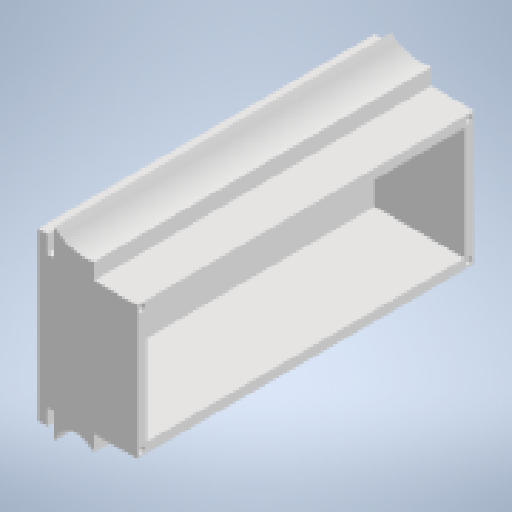
# Autodesk Inventor part: Casing
Saved by Autodesk Inventor 2025.2 (Build 292293000, 293)
## iProperties
Created: 2025-01-21
Part Number: Casing
Material: Generic
Document SubType Name: Modeling
Designer: armenanzasn25
Density: 1 g/cm^3
Appearance: Default
TUBE_OUTER: 0.545 in
Author: armenanzasn25
Autodesk Inventor part; units mm, degrees
ref_plane "YZ Plane" through (0, 0, 0) normal (1, 0, 0) x (0, 1, 0)
ref_plane "XZ Plane" through (0, 0, 0) normal (0, 1, 0) x (-1, 0, 0)
ref_plane "XY Plane" through (0, 0, 0) normal (0, 0, 1) x (1, 0, 0)
sketch "Sketch2" plane through (0, 0, 0) normal (0, 0, 1) x (1, 0, 0)
  line L0 (-3, 8) -> (-3, -48)
  line L1 (-3, 8) -> (3, 8)
  line L2 (3, 8) -> (3, 3)
  line L3 (3, 3) -> (5, 3)
  line L4 (5, 3) -> (5, 10.4583)
  arc A0 (5, 10.4583) -> (17, 10.4583) centre (11, 13.909) ccw
  line L5 (17, 10.4583) -> (17, 3)
  line L6 (17, 3) -> (27, 3)
  line L7 (-3, -48) -> (3, -48)
  line L8 (3, -43) -> (3, -48)
  line L9 (27, -43) -> (17, -43)
  arc A1 (17, -50.4583) -> (5, -50.4583) centre (11, -53.909) ccw
  line L10 (3, -43) -> (5, -43)
  line L11 (5, -43) -> (5, -50.4583)
  line L12 (17, -43) -> (17, -50.4583)
  line L13 (27, 3) -> (27, 0)
  line L14 (27, 0) -> (0, 0)
  line L15 (0, 0) -> (0, -40)
  line L16 (0, -40) -> (27, -40)
  line L17 (27, -40) -> (27, -43)
  dimension "d13" = 12
  dimension "d14" = 2
  dimension "d20" = 5
  dimension "d22" = 13.843
  dimension "d29" = 3
  dimension "d30" = 3
  dimension "d31" = 3
  dimension "d33" = 40
  dimension "d34" = 27
  dimension "d36" = 16
  dimension "d38" = 67.818
  dimension "d53" = 6.9215
  dimension "d54" = 10
  constraints: 36 end point, 8 perpendicular, 5 equal length, 4 point on circle, 4 vertical, 3 horizontal, 2 centre point, 2 collinear, 2 point on line, 1 coincident, 1 vertical alignment
  measures "d13" distance between parallel lines of L5 L4
  measures "d14" distance of L2.end L3.end
  measures "d20" distance between parallel lines of L1 L3
  measures "d22" diameter of A1
  measures "d29" distance between parallel lines of L6 L14
  measures "d30" distance between parallel lines of L0 L15
  measures "d31" distance between parallel lines of L9 L16
  measures "d33" distance between parallel lines of L16 L14
  measures "d34" distance of L13.end L14.end
  measures "d36" distance from line of L13 A0.centre
  measures "d38" distance of A1.centre A0.centre
  measures "d53" radius of A0
  measures "d54" distance between parallel lines of L13 L5
extrude "Extrusion1" add sketch "Sketch2" along normal blind 101.6
sketch "Sketch3" plane through (0, -40, 0) normal (1, 0, 0) x (0, 0, -1)
  line L0 (0, 0) -> (0, 40) projected
  line L1 (0, 40) -> (-101.6, 40) projected
  line L2 (-101.6, 0) -> (-101.6, 40) projected
  line L3 (0, 0) -> (-101.6, 0) projected
  line L4 (-101.6, 40) -> (-98.6, 40)
  line L5 (-98.6, 40) -> (-98.6, 0)
  line L6 (-98.6, 0) -> (-101.6, 0)
  line L7 (-101.6, 0) -> (-101.6, 40)
  line L8 (0, 40) -> (-3, 40)
  line L9 (-3, 40) -> (-3, 0)
  line L10 (-3, 0) -> (0, 0)
  line L11 (0, 0) -> (0, 40)
  dimension "d39" = 3
  dimension "d40" = 3
  constraints: 16 end point, 4 parallel, 2 horizontal, 2 perpendicular, 2 point on line
  measures "d39" distance between parallel lines of L5 L2
  measures "d40" distance between parallel lines of L0 L9
extrude "Extrusion2" add sketch "Sketch3" along normal blind 27 contours L3 L9 L1 L0 | L3 L2 L1 L5
sketch "Sketch4" plane through (27, -43, 0) normal (1, 0, 0) x (0, 0, -1)
  circle A0 centre (-100.1, 44.5) radius 1
  line L0 (-3, 3) -> (-98.6, 3) projected
  line L1 (-98.6, 3) -> (-98.6, 43) projected
  line L2 (-3, 43) -> (-98.6, 43) projected
  line L3 (-3, 43) -> (-3, 3) projected
  line L4 (0, 0) -> (0, 46) projected
  line L5 (0, 46) -> (-101.6, 46) projected
  line L6 (-101.6, 0) -> (-101.6, 46) projected
  line L7 (0, 0) -> (-101.6, 0) projected
  circle A1 centre (-1.5, 44.5) radius 1
  circle A2 centre (-1.5, 1.5) radius 1
  circle A3 centre (-100.1, 1.5) radius 1
  point P0 (0, 43)
  dimension "d43" = 2
  dimension "d44" = 1.5
  dimension "d45" = 1.5
  dimension "d47" = 1.5
  dimension "d48" = 1.5
  constraints: 4 centre point, 3 equal radius, 2 horizontal alignment, 2 vertical alignment
  measures "d43" diameter of A0
  measures "d44" distance from line of L5 A0.centre
  measures "d45" distance from line of L6 A0.centre
  measures "d47" distance from line of L7 A2.centre
  measures "d48" distance from line of L4 A2.centre
extrude "Extrusion3" cut sketch "Sketch4" against normal blind 10 contours A0 | A1 | A2 | A3
equation "\"TUBE_OUTER\" = 13.843"
equation "\"INTER_TUBE\" = 53.975"
equation "\"CUPPING\" = 5.08"
equation "\"d19\" = TUBE_OUTER"
equation "\"W_THICK\" = 3"
equation "\"SCREW_D\" = 2"
body "Solid1"
